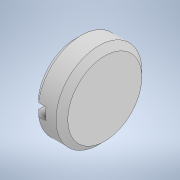
# Autodesk Inventor part: 711113
Saved by Autodesk Inventor 2022 (Build 260153000, 153)
## iProperties
Created: 2021-10-21
Part Number: 711113
Material: Типовые
Document SubType Name: Modeling
Designer: RaNSiD
Density: 1 g/cm^3
Appearance: По умолчанию
Author: RaNSiD
Autodesk Inventor part; units mm, degrees
ref_plane "YZ Plane" through (0, 0, 0) normal (1, 0, 0) x (0, 1, 0)
ref_plane "XZ Plane" through (0, 0, 0) normal (0, 1, 0) x (-1, 0, 0)
ref_plane "XY Plane" through (0, 0, 0) normal (0, 0, 1) x (1, 0, 0)
sketch "Эскиз1" plane through (0, 0, 0) normal (0, 0, 1) x (1, 0, 0)
  line L0 (0, 0) -> (20, 0)
  line L1 (20, 0) -> (20, 25)
  line L2 (16, 29) -> (4, 29)
  line L3 (0, 25) -> (0, 0)
  line L4 (4, 29) -> (0, 25)
  line L5 (16, 29) -> (20, 25)
  point P0 (20, 29)
  point P1 (0, 29)
  dimension "d12" = 20
  dimension "d13" = 29
  dimension "d14" = 4
  dimension "d15" = 4
  dimension "d16" = 4
  dimension "d17" = 4
  constraints: 12 end point, 4 point on line, 2 parallel, 1 horizontal, 1 perpendicular
  measures "d12" distance of point (0, 29) point (20, 29)
  measures "d13" distance of point (20, 29) L0.end
  measures "d14" distance of L2.end point (0, 29)
  measures "d15" distance of L3.start point (0, 29)
  measures "d16" distance of L2.start point (20, 29)
  measures "d17" distance of L1.end point (20, 29)
revolve "Вращение2" add sketch "Эскиз1" angle 360 about axis through (0, 0, 0) along (1, 0, 0)
sketch "Эскиз4" plane through (0, 0, 0) normal (0, 0, 1) x (1, 0, 0)
  line L0 (0, -25) -> (0, 25) construction
  line L1 (0, 4) -> (9, 4)
  line L2 (9, 4) -> (9, -4)
  line L3 (9, -4) -> (0, -4)
  line L4 (0, -4) -> (0, 4)
  point P0 (0, 0)
  point P1 (0, 0)
  point P2 (0, 0)
  dimension "d23" = 9
  dimension "d24" = 8
  constraints: 8 end point, 2 midpoint, 2 parallel, 1 coincident, 1 horizontal, 1 perpendicular, 1 point on line
  measures "d23" distance of L2.end L3.end
  measures "d24" distance of L1.end L2.end
extrude "Выдавливание3" cut sketch "Эскиз4" along normal through all both and the other way through all
equation "\"d15\" = d14"
equation "\"d16\" = d14"
equation "\"d17\" = d16"
